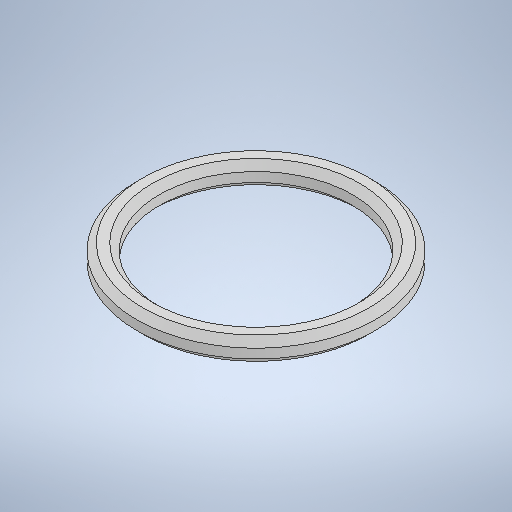
# Autodesk Inventor part: Ring
Saved by Autodesk Inventor 2026.2 (Build 302298010, 298A)
## iProperties
Created: 2026-05-02
Part Number: Ring
Material: Generic
Document SubType Name: Modeling
Designer: piete
Density: 1 g/cm^3
Appearance: Default
Author: piete
Autodesk Inventor part; units mm, degrees
ref_plane "YZ Plane" through (0, 0, 0) normal (1, 0, 0) x (0, 1, 0)
ref_plane "XZ Plane" through (0, 0, 0) normal (0, 1, 0) x (-1, 0, 0)
ref_plane "XY Plane" through (0, 0, 0) normal (0, 0, 1) x (1, 0, 0)
sketch "Sketch1" plane through (0, 0, 0) normal (1, 0, 0) x (0, 1, 0)
  line L0 (-0.4142, 8.5) -> (-1, 9.0858)
  line L1 (-1, 9.0858) -> (-1, 9.9142)
  line L2 (-1, 9.9142) -> (-0.4142, 10.5)
  line L3 (-0.4142, 10.5) -> (0.4142, 10.5)
  line L4 (0.4142, 10.5) -> (1, 9.9142)
  line L5 (1, 9.9142) -> (1, 9.0858)
  line L6 (1, 9.0858) -> (0.4142, 8.5)
  line L7 (0.4142, 8.5) -> (-0.4142, 8.5)
  line L8 (3.1428, 0) -> (-2.1354, 0)
  point P0 (0, 0)
  point P1 (0, 9.5)
  dimension "d2" = 2
  dimension "d3" = 0
  dimension "d5" = 8.5
  constraints: 18 end point, 2 horizontal, 17 other
  measures "d2" distance between parallel lines of L1 L5
  measures "d3" horizontal distance of point (0, 0) point (0, 9.5)
  measures "d5" distance from line of point (0, 0) L7
revolve "Revolution1" add sketch "Sketch1" angle 360 about axis through (0, 3.1428, 0) along (0, -1, 0)
body "Solid1"
